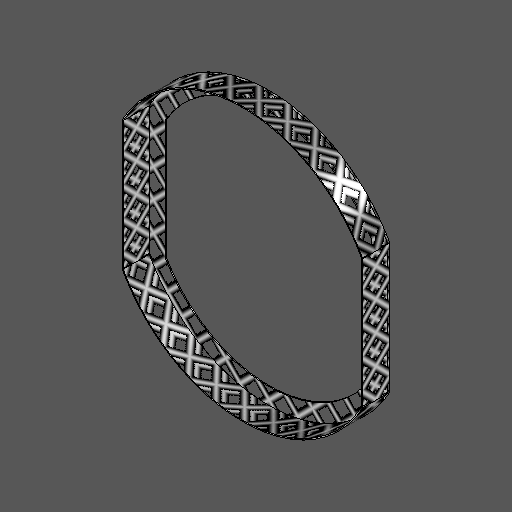
# Autodesk Inventor part: probe-gate-mesh
Saved by Autodesk Inventor 2025 (Build 290162000, 162)
## iProperties
Created: 2024-05-16
Part Number: probe-gate-mesh
Material: Stainless Steel
Document SubType Name: Modeling
Designer: kuzmin
Density: 8 g/cm^3
Appearance: Expanded Metal 02
Author: kuzmin
Autodesk Inventor part; units mm, degrees
ref_plane "YZ Plane" through (0, 0, 0) normal (1, 0, 0) x (0, 1, 0)
ref_plane "XZ Plane" through (0, 0, 0) normal (0, 1, 0) x (-1, 0, 0)
ref_plane "XY Plane" through (0, 0, 0) normal (0, 0, 1) x (1, 0, 0)
sketch "Sketch1" plane through (0, 0, 0) normal (0, 0, 1) x (1, 0, 0)
  arc A0 (22, 11.8743) -> (-22, 11.8743) centre (0, 0) ccw
  arc A1 (-22, -11.8743) -> (22, -11.8743) centre (0, 0) ccw
  line L0 (-22, 11.8743) -> (-22, -11.8743)
  line L1 (22, -11.8743) -> (22, 11.8743)
  line L2 (-22.2, 11.9248) -> (-22.2, -11.9248)
  arc A2 (-22.2, -11.9248) -> (22.2, -11.9248) centre (0, 0) ccw
  line L3 (22.2, -11.9248) -> (22.2, 11.9248)
  arc A3 (22.2, 11.9248) -> (-22.2, 11.9248) centre (0, 0) ccw
  line L4 (-19, 11.0905) -> (-19, -11.0905)
  arc A4 (-19, -11.0905) -> (19, -11.0905) centre (0, 0) ccw
  line L5 (19, -11.0905) -> (19, 11.0905)
  arc A5 (19, 11.0905) -> (-19, 11.0905) centre (0, 0) ccw
  point P0 (-22, 0)
  point P1 (22, 0)
  dimension "d1" = 44
  dimension "d2" = 50
  dimension "d3" = 3
  dimension "d4" = 0.2
  constraints: 12 end point, 12 point on circle, 6 centre point, 3 horizontal alignment, 2 coincident, 2 midpoint, 2 vertical, 6 other
  measures "d1" distance between parallel lines of L1 L0
  measures "d2" diameter of A0
  measures "d3" distance between parallel lines of L1 L5
  measures "d4" distance between parallel lines of L3 L1
extrude "Extrusion1" add sketch "Sketch1" along normal blind 0.2 contours L1 A1 L0 A0
extrude "Extrusion2" add sketch "Sketch1" along normal blind 5 contours A3 L3 A2 L2
equation "\"d4\" = thickness"
equation "\"d5\" = thickness"
equation "\"thickness\" = 0.2"
body "Solid1"
